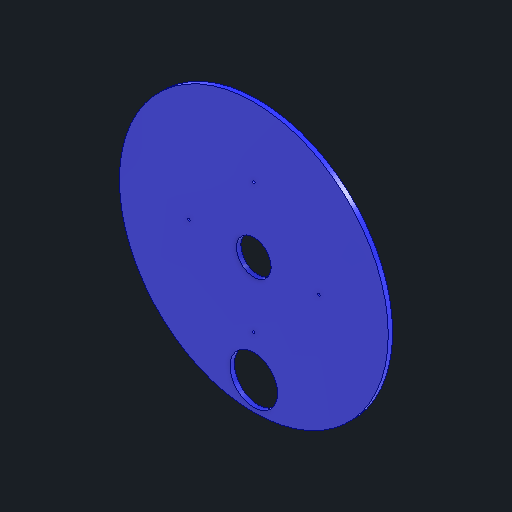
# Autodesk Inventor part: Part1
Saved by Autodesk Inventor 2027.1 (Build 311270010, 270A)
## iProperties
Created: 2026-09-28
Part Number: Part1
Material: Steel, Paint Finish, Blue
Document SubType Name: Modeling
Designer: daniel
Density: 7.85 g/cm^3
Appearance: Blue - Wall Paint - Glossy
Mass: 2574.04 g
Surface Area: 1387.01 cm^2
Volume: 327.904 cm^3
Author: daniel
Autodesk Inventor part; units mm, degrees
ref_plane "YZ Plane" through (0, 0, 0) normal (1, 0, 0) x (0, 1, 0)
ref_plane "XZ Plane" through (0, 0, 0) normal (0, 1, 0) x (-1, 0, 0)
ref_plane "XY Plane" through (0, 0, 0) normal (0, 0, 1) x (1, 0, 0)
sketch "Sketch1" plane through (0, 0, 0) normal (0, 0, 1) x (1, 0, 0)
  circle A0 centre (0, 0) radius 150
  circle A1 centre (0, 0) radius 155
  circle A2 centre (0, -122.5) radius 27.5
  circle A3 centre (0, 0) radius 87.5
  circle A4 centre (0, 0) radius 75
  circle A5 centre (0, 0) radius 50
  circle A6 centre (75, 0) radius 1.5
  circle A7 centre (0, -75) radius 1.5
  circle A8 centre (0, 75) radius 1.5
  circle A9 centre (-75, 0) radius 1.5
  circle A10 centre (0, 0) radius 20
  point P0 (0, -150)
  dimension "d0" = 300
  dimension "d2" = 310
  dimension "d3" = 55
  dimension "d8" = 175
  dimension "d9" = 150
  dimension "d10" = 100
  dimension "d11" = 3
  dimension "d12" = 3
  dimension "d13" = 3
  dimension "d14" = 3
  dimension "d15" = 40
  constraints: 11 centre point, 5 coincident, 4 point on circle, 1 tangent
  measures "d0" diameter of A0
  measures "d2" diameter of A1
  measures "d3" diameter of A2
  measures "d8" diameter of A3
  measures "d9" diameter of A4
  measures "d10" diameter of A5
  measures "d11" diameter of A6
  measures "d12" diameter of A7
  measures "d13" diameter of A8
  measures "d14" diameter of A9
  measures "d15" diameter of A10
extrude "Extrusion1" add sketch "Sketch1" along normal blind 5 contours A0 | A1 | A3 | A6 A4 A7 A9 A8 | A5
equation "\"d0\" = 6 * Product_dia"
equation "\"d8\" = 3.5 * Product_dia"
equation "\"d12\" = d11"
equation "\"d13\" = d11"
equation "\"d14\" = d11"
equation "\"GridTotalSize\" = 65"
equation "\"GridBorderThickness\" = 5"
equation "\"AluminiumExtrusionClearance\" = 35"
equation "\"GridRobotClearance\" = 65"
equation "\"GridBorderFillets\" = 7"
equation "\"GridProcutClearance\" = 5"
equation "\"WorkspaceLength\" = 515"
equation "\"AxesBaseFillet\" = 15"
equation "\"ProductTotalHeight\" = 45"
equation "\"VerticalStroke\" = 105"
equation "\"Zaxis\" = 197"
equation "\"WorkspaceHeight\" = 183"
equation "\"BaseTotalLength\" = 885"
equation "\"BackArea\" = 165"
equation "\"CylinderStroke\" = 75"
equation "\"BoxesWidth\" = 125"
equation "\"BaseWoodThickness\" = 7"
equation "\"kerf\" = 1.5"
equation "\"Kerf\" = 0.3"
equation "\"RxThickness\" = 1.8"
equation "\"Product_dia\" = 50"
body "Solid1"
